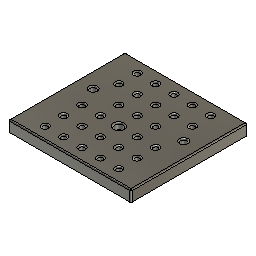
camera_holder v1 (Autodesk Fusion 360 design; units mm, degrees)
Autodesk Fusion 360 part; units mm, degrees
sketch "Sketch1" plane through (0, 0, 0) normal (0, 0, 1) x (1, 0, 0)
  line L0 (0, 0) -> (100, 0)
  line L1 (100, 0) -> (100, 95)
  line L2 (100, 95) -> (0, 95)
  line L3 (0, 95) -> (0, 0)
  circle A0 centre (20, 85) radius 2
  line L4 (50, 95) -> (50, 0) construction
  line L5 (0, 47.5) -> (100, 47.5) construction
  circle A1 centre (35, 85) radius 2
  circle A2 centre (50, 85) radius 2
  circle A3 centre (65, 85) radius 2
  circle A4 centre (80, 85) radius 2
  circle A5 centre (20, 70) radius 2
  circle A6 centre (35, 70) radius 2
  circle A7 centre (50, 70) radius 2
  circle A8 centre (65, 70) radius 2
  circle A9 centre (80, 70) radius 2
  circle A10 centre (35, 55) radius 2
  circle A11 centre (50, 55) radius 2
  circle A12 centre (65, 55) radius 2
  circle A13 centre (20, 40) radius 2
  circle A14 centre (35, 40) radius 2
  circle A15 centre (65, 40) radius 2
  circle A16 centre (80, 40) radius 2
  circle A17 centre (20, 25) radius 2
  circle A18 centre (35, 25) radius 2
  circle A19 centre (50, 25) radius 2
  circle A20 centre (65, 25) radius 2
  circle A21 centre (80, 25) radius 2
  circle A22 centre (20, 10) radius 2
  circle A23 centre (35, 10) radius 2
  circle A24 centre (50, 10) radius 2
  circle A25 centre (65, 10) radius 2
  circle A26 centre (80, 10) radius 2
  circle A27 centre (13, 56) radius 2.5
  circle A28 centre (87, 56) radius 2.5
  circle A29 centre (50, 40) radius 3.5
  dimension "d1" = 100
  dimension "d2" = 95
  dimension "d3" = 4
  dimension "d10" = 60
  dimension "d11" = -75
  dimension "d12" = 10
  dimension "d13" = 20
  dimension "d14" = 5
  dimension "d15" = 5
  dimension "d16" = 7
  dimension "d17" = 16
  dimension "d18" = 74
  dimension "d19" = 37
  constraint horizontal L0
  constraint vertical L1
  constraint horizontal L2
  constraint vertical L3
  constraint coincident L0.start L3.end
  constraint midpoint L2 L4.start
  constraint midpoint L0 L4.end
  constraint midpoint L3 L5.start
  constraint midpoint L1 L5.end
  constraint coincident L4 A29.centre
  constraint horizontal A27.centre A28.centre
  constraint horizontal A14.centre A29.centre
  measures "d1" distance of L1.end L2.end
  measures "d2" distance of L0.start L2.end
  measures "d3" diameter of A0
  measures "d12" distance of L2 A0.centre
  measures "d13" distance of L3 A0.centre
  measures "d14" diameter of A27
  measures "d15" diameter of A28
  measures "d16" diameter of A29
  measures "d17" vertical distance of A28.centre A29.centre
  measures "d18" distance of A27.centre A28.centre
  measures "d19" distance of L4 A27.centre
extrude "Extrude1" add sketch "Sketch1" along normal blind 10
sketch "Sketch2" plane through (0, 0, 0) normal (0, 0, -1) x (1, 0, 0)
  circle A0 centre (35, -85) radius 2
  circle A1 centre (50, -55) radius 2
  circle A2 centre (20, -85) radius 2
  circle A3 centre (80, -85) radius 2
  circle A4 centre (65, -85) radius 2
  circle A5 centre (50, -85) radius 2
  circle A6 centre (35, -55) radius 2
  circle A7 centre (80, -70) radius 2
  circle A8 centre (65, -70) radius 2
  circle A9 centre (50, -70) radius 2
  circle A10 centre (35, -70) radius 2
  circle A11 centre (20, -70) radius 2
  circle A12 centre (65, -55) radius 2
  circle A13 centre (20, -40) radius 2
  circle A14 centre (35, -40) radius 2
  circle A15 centre (65, -40) radius 2
  circle A16 centre (80, -40) radius 2
  circle A17 centre (20, -25) radius 2
  circle A18 centre (35, -25) radius 2
  circle A19 centre (50, -25) radius 2
  circle A20 centre (65, -25) radius 2
  circle A21 centre (80, -25) radius 2
  circle A22 centre (20, -10) radius 2
  circle A23 centre (35, -10) radius 2
  circle A24 centre (50, -10) radius 2
  circle A25 centre (65, -10) radius 2
  circle A26 centre (80, -10) radius 2
  circle A27 centre (13, -56) radius 2.5
  circle A28 centre (87, -56) radius 2.5
  circle A29 centre (50, -40) radius 3.5
  line L0 (0, 0) -> (0, -95)
  line L1 (0, -95) -> (100, -95)
  line L2 (100, -95) -> (100, 0)
  line L3 (100, 0) -> (0, 0)
  circle A30 centre (50, -40) radius 7.5
  circle A31 centre (87, -56) radius 5
  circle A32 centre (13, -56) radius 5
  dimension "d22" = 10
  dimension "d23" = 10
  dimension "d24" = 15
  constraint concentric A29 A30
  constraint concentric A28 A31
  constraint concentric A27 A32
  measures "d22" diameter of A31
  measures "d23" diameter of A32
  measures "d24" diameter of A30
extrude "Extrude2" cut sketch "Sketch2" against normal blind 5 contours A30 | A31 | A32
fillet "Fillet1" radius 1 1 edges at (8.3384, 54.1919, 0) 6 faces at (90.881, 25.9657, 0) (90.3478, 26.6299, 10) (33.3333, 0, 3.3333) (100, 31.6667, 3.3333) (66.6667, 95, 3.3333) (0, 63.3333, 3.3333)
equation "d19 = ( 74 / 2 ) * 1 mm"
